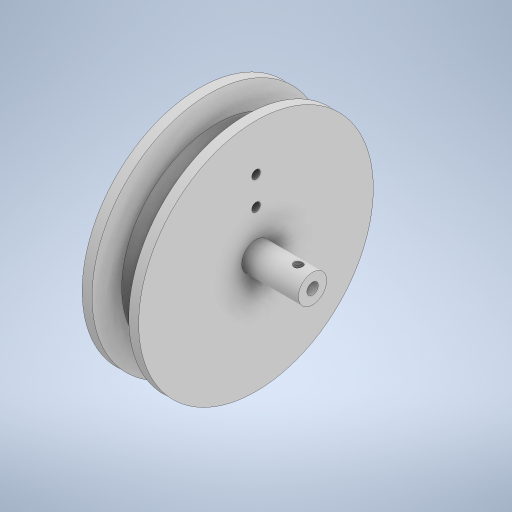
# Autodesk Inventor part: Шкив 80
Saved by Autodesk Inventor 2023 (Build 270158000, 158)
## iProperties
Created: 2022-05-01
Part Number: Шкив 80
Material: Типовые
Document SubType Name: Modeling
Designer: User
Density: 1 g/cm^3
Appearance: По умолчанию
Author: User
Autodesk Inventor part; units mm, degrees
ref_plane "YZ Plane" through (0, 0, 0) normal (1, 0, 0) x (0, 1, 0)
ref_plane "XZ Plane" through (0, 0, 0) normal (0, 1, 0) x (-1, 0, 0)
ref_plane "XY Plane" through (0, 0, 0) normal (0, 0, 1) x (1, 0, 0)
sketch "Эскиз1" plane through (0, 0, 0) normal (0, 1, 0) x (-1, 0, 0)
  line L0 (0, 0) -> (20, 0)
  line L1 (20, 0) -> (20, 41.5)
  line L2 (20, 41.5) -> (0, 41.5)
  line L3 (0, 41.5) -> (0, 0)
  line L4 (20, 41.5) -> (14, 41.5)
  line L5 (14, 41.5) -> (14, 33.5)
  line L6 (14, 33.5) -> (6, 33.5)
  line L7 (6, 33.5) -> (6, 41.5)
  line L8 (10, 33.5) -> (10, 41.5)
  line L9 (10, 41.5) -> (3.5, 41.5)
  line L10 (3.5, 41.5) -> (6, 33.5)
  line L11 (10, 41.5) -> (16.5, 41.5)
  line L12 (16.5, 41.5) -> (14, 33.5)
  dimension "d0" = 20
  dimension "d1" = 41.5
  dimension "d2" = 6
  dimension "d3" = 8
  dimension "d4" = 8
  dimension "d38" = 6.5
  dimension "d39" = 6.5
  constraints: 26 end point, 6 perpendicular, 4 point on line, 2 midpoint, 1 horizontal
  measures "d0" distance of L0.start L0.end
  measures "d1" distance of L0.end L1.end
  measures "d2" distance of L1.end L4.end
  measures "d3" distance of L4.end L5.end
  measures "d4" distance of L5.end L6.end
  measures "d38" distance of L8.end L9.end
  measures "d39" distance of L8.end L11.end
revolve "Вращение1" add sketch "Эскиз1" angle 360 about axis through (0, 0, 0) along (-1, 0, 0) contours L3 L2 L10 L6 L12 L1 L0
sketch "Эскиз2" plane through (0, 0, 0) normal (1, 0, 0) x (0, 0, -1)
  circle A0 centre (0, 0) radius 5
  dimension "d6" = 10
  constraints: 1 centre point, 1 coincident
  measures "d6" diameter of A0
extrude "Выдавливание1" add sketch "Эскиз2" along normal blind 20
sketch "Эскиз3" plane through (20, 0, 0) normal (1, 0, 0) x (0, 0, -1)
  circle A0 centre (0, 0) radius 2
  dimension "d9" = 4
  constraints: 1 centre point, 1 coincident
  measures "d9" diameter of A0
extrude "Выдавливание2" cut sketch "Эскиз3" against normal blind 20
sketch "Эскиз4" plane through (0, 0, 0) normal (1, 0, 0) x (0, 0, -1)
  circle A0 centre (0, 0) radius 5 projected
  point P0 (0, 5)
  constraints: 1 vertical alignment, 1 other
ref_plane "РабПлоскость1" through (0, 5, 0) normal (0, 1, 0) x (-1, 0, 0)
sketch "Эскиз5" plane through (0, 5, 0) normal (0, 1, 0) x (-1, 0, 0)
  line L0 (0, 0) -> (-15, 0)
  circle A0 centre (-15, 0) radius 1.5
  dimension "d18" = 15
  dimension "d19" = 3
  constraints: 2 end point, 1 centre point, 1 coincident, 1 horizontal
  measures "d18" distance of L0.start L0.end
  measures "d19" diameter of A0
extrude "Выдавливание3" cut sketch "Эскиз5" against normal blind 58
thread "Резьба1" size "M3x0.5" class "6H" standard "ISO Metric profile" full length
ref_plane "РабПлоскость2" through (-10, 0, 0) normal (-1, 0, 0) x (0, 0, 1)
sketch "Эскиз6" plane through (0, 0, 0) normal (1, 0, 0) x (0, 0, -1)
  circle A0 centre (0, 0) radius 5 projected
  line L0 (0, 0) -> (0, 25)
  circle A1 centre (0, 25) radius 1.5
  line L1 (0, 0) -> (0, 15)
  circle A2 centre (0, 15) radius 1.5
  dimension "d28" = 25
  dimension "d29" = 3
  dimension "d42" = 15
  dimension "d43" = 3
  constraints: 4 end point, 2 centre point, 2 coincident, 1 point on line, 1 vertical
  measures "d28" distance of L0.start L0.end
  measures "d29" diameter of A1
  measures "d42" distance of L0.start L1.end
  measures "d43" diameter of A2
extrude "Выдавливание4" cut sketch "Эскиз6" against normal blind 59.75 contours A2 L0 | L0 A2 | A1
thread "Резьба2" size "M3x0.5" class "6H" standard "ANSI Metric M Profile" full length
thread "Резьба3" size "M3x0.5" class "6H" standard "ANSI Metric M Profile" full length
